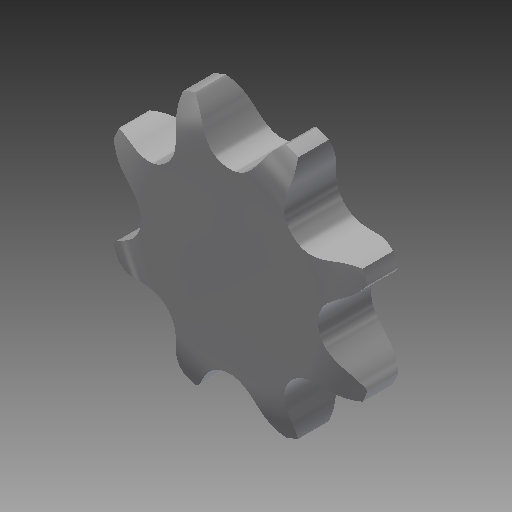
# Autodesk Inventor part: Roller Chain Sprocket1
Saved by Autodesk Inventor 2017 (Build 210142000, 142)
## iProperties
Created: 2016-10-04
Part Number: Roller Chain Sprocket1
Material: Steel
Document SubType Name: Modeling
Designer: hanso
Density: 1 g/cm^3
Appearance: Steel
CustomPartVersion: 1
Author: hanso
Autodesk Inventor part; units mm, degrees
ref_plane "YZ Plane" through (0, 0, 0) normal (1, 0, 0) x (0, 1, 0)
ref_plane "XZ Plane" through (0, 0, 0) normal (0, 1, 0) x (-1, 0, 0)
sketch "Theoretical Tooth Profile" plane through (0, 0, 0) normal (0, 0, 1) x (1, 0, 0)
  circle A0 centre (0, 0) radius 16.5933 construction
  line L0 (0, 0) -> (0, 16.5933) construction
  line L1 (0, 0) -> (11.7333, 11.7333) construction
  circle A1 centre (0, 0) radius 19.1403
  arc A2 (-2.9641, 13.8773) -> (2.9641, 13.8773) centre (0, 16.5933) ccw
  line L2 (0, 16.5933) -> (11.7333, 11.7333) construction
  line L3 (0, 16.5933) -> (4.6742, 20.8765) construction
  line L4 (4.6742, 20.8765) -> (-4.1593, 15.4633) construction
  arc A3 (6.4582, 18.0178) -> (4.434, 15.9117) centre (10.2502, 12.3476) ccw
  arc A4 (-4.434, 15.9117) -> (-6.4582, 18.0178) centre (-10.2502, 12.3476) ccw
  line L5 (-10.2502, 12.3476) -> (-4.434, 15.9117) construction
  arc A5 (-4.1593, 15.4633) -> (-2.9641, 13.8773) centre (4.6742, 20.8765) ccw
  line L6 (-4.1593, 15.4633) -> (-4.434, 15.9117)
  arc A6 (2.9641, 13.8773) -> (4.1593, 15.4633) centre (-4.6742, 20.8765) ccw
  line L7 (4.434, 15.9117) -> (4.1593, 15.4633)
  line L8 (0, 0) -> (7.3247, 17.6833) construction
  point P0 (5.8666, 14.1633)
  dimension "d0" = 33.1867
  dimension "d2" = 45
  dimension "d3" = 4.0203
  dimension "d10" = 132.5
  dimension "d11" = 11
  dimension "d12" = 6.3398
  dimension "d13" = 10.3602
  dimension "d14" = 11.0947
  dimension "d23" = 3.81
  constraints: 18 end point, 15 point on circle, 7 centre point, 3 coincident, 3 point on line, 3 symmetric about line, 3 tangent, 1 equal radius, 1 midpoint, 1 parallel, 1 vertical, 1 other
  measures "d0" diameter of A0
  measures "d2" angle of L1 L0
  measures "d3" radius of A2
  measures "d10" angle of L3 L0
  measures "d11" angle of L4 L3
  measures "d12" distance of L2.start L3.end
  measures "d13" distance of L3.end L4.end
  measures "d14" distance of A3.centre L0.end
  measures "d23" distance from line of L8.end L2
sketch "Tooth Profile" plane through (0, 0, 0) normal (0, 0, 1) x (1, 0, 0)
  circle A0 centre (0, 0) radius 19.1403 projected
  line L0 (0, 0) -> (0, 16.5933) construction
  line L1 (0, 16.5933) -> (3.6249, 14.8546) construction
  arc A1 (-3.6249, 14.8546) -> (3.6249, 14.8546) centre (0, 16.5933) ccw
  line L2 (-3.6249, 14.8546) -> (0, 16.5933) construction
  arc A2 (-3.6249, 14.8546) -> (-6.1894, 18.1119) centre (-12.1993, 10.7419) ccw
  arc A3 (6.1894, 18.1119) -> (3.6249, 14.8546) centre (12.1993, 10.7419) ccw
  dimension "d44" = 128.75
  dimension "d45" = 4.0203
  dimension "d46" = 9.5098
  constraints: 8 point on circle, 7 end point, 3 centre point, 2 tangent, 1 coincident, 1 equal radius, 1 symmetric about line, 1 vertical
  measures "d44" angle of L1 L2
  measures "d45" radius of A1
  measures "d46" radius of A3
sketch "Section Profile" plane through (0, 0, 0) normal (1, 0, 0) x (0, 1, 0)
  line L0 (19.1403, 0) -> (-19.1403, 0) projected
  line L1 (8.0913, 3.7612) -> (-8.0913, 3.7612)
  line L2 (-8.0913, 3.7612) -> (-8.0913, -3.7612)
  line L3 (-8.0913, -3.7612) -> (8.0913, -3.7612)
  line L4 (8.0913, -3.7612) -> (8.0913, 3.7612)
  line L5 (8.0913, 3.7612) -> (19.1403, 3.7612) construction
  line L6 (19.1403, 3.7612) -> (19.1403, -3.7612) construction
  line L7 (19.1403, -3.7612) -> (8.0913, -3.7612) construction
  line L8 (8.0913, -3.7612) -> (8.0913, 3.7612)
  arc A0 (19.1403, 2.1737) -> (12.7887, 3.7612) centre (12.7887, -9.7389) ccw
  arc A1 (12.7887, -3.7612) -> (19.1403, -2.1737) centre (12.7887, 9.7389) ccw
  line L9 (12.7887, 3.7612) -> (0, 3.7612)
  line L10 (0, 3.7612) -> (0, -3.7612)
  line L11 (0, -3.7612) -> (12.7887, -3.7612)
  line L12 (0, 3.7612) -> (0, -3.7612)
  line L13 (19.1403, 2.1737) -> (19.1403, -2.1737)
  point P0 (0, 0)
  point P1 (0, 0)
  dimension "d30" = 7.5225
  dimension "d31" = 16.1825
  dimension "d32" = 7.5225
  dimension "d33" = 1.5875
  dimension "d34" = 13.5001
  dimension "d43" = 3.7612
  constraints: 26 end point, 7 midpoint, 5 perpendicular, 4 parallel, 4 point on circle, 3 point on line, 3 symmetric about line, 2 centre point, 2 horizontal, 2 tangent, 1 collinear, 1 other
  measures "d30" distance between parallel lines of L7 L5
  measures "d31" distance between parallel lines of L2 L4
  measures "d32" distance between parallel lines of L3 L1
  measures "d33" distance from line of L13.start L5
  measures "d34" radius of A0
  measures "d43" distance between parallel lines of L3 L0
revolve "Shroud" add sketch "Section Profile" angle 360 about axis through (0, 0, 3.7612) along (0, 0, -1) contours L10 L3 L2 L0 | L0 L2 L1 L10
revolve "Strand" add sketch "Section Profile" angle 360 about axis through (0, 0, 3.7612) along (0, 0, -1) contours L13 A1 L11 L4 L0 | L0 L4 L9 A0 L13 | L4 L3 L10 L0 | L0 L10 L1 L4
pattern_of_one "Strand Pattern"
extrude "Theoretical Tooth" cut sketch "Theoretical Tooth Profile" along normal through all both and the other way through all contours A3 L7 A6 A2 A5 L6 A4 A1 picked at (0.1583, 16.8767)
extrude "Tooth" [suppressed]
pattern_circular "Tooth Pattern" count 8 over 360 about axis through (0, 0, -10) along (0, 0, 1) of "Theoretical Tooth"
ref_plane "Timing Plane" through (0, 16.5933, 0) normal (1, 0, 0) x (0, 1, 0)
equation "\"d3\" = 0.5 * da_Dr + da_SC"
equation "\"d12\" = 0.8 * da_Dr"
equation "\"d13\" = 1.3 * da_Dr + da_SC"
equation "\"d14\" = 1.4 * da_Dr"
equation "\"d23\" = da_Ha"
equation "\"d44\" = da_Alfa"
equation "\"d45\" = da_Ri"
equation "\"d46\" = da_Re"
equation "\"d30\" = da_Bf"
equation "\"d31\" = da_Ds"
equation "\"d32\" = da_Bs"
equation "\"d33\" = da_Ba"
equation "\"d34\" = da_Rx"
equation "\"d40\" = da_pt"
equation "\"form_type\" = 0"
equation "\"da_p\" = 12.7"
equation "\"da_Dr\" = 7.9248"
equation "\"da_SC\" = 0.05791"
equation "\"da_Ha\" = 3.81"
equation "\"da_pt\" = 14.3764"
equation "\"da_Bf\" = 7.52246"
equation "\"da_Ba\" = 1.5875"
equation "\"da_Rx\" = 13.5001"
equation "\"da_Ra\" = 0.508"
equation "\"da_Bs\" = 7.52246"
equation "\"da_Ds\" = 16.18251"
equation "\"da_Re\" = 9.50976"
equation "\"da_Ri\" = 4.02031"
equation "\"da_Alfa\" = 128.75deg"
body "Solid1"
